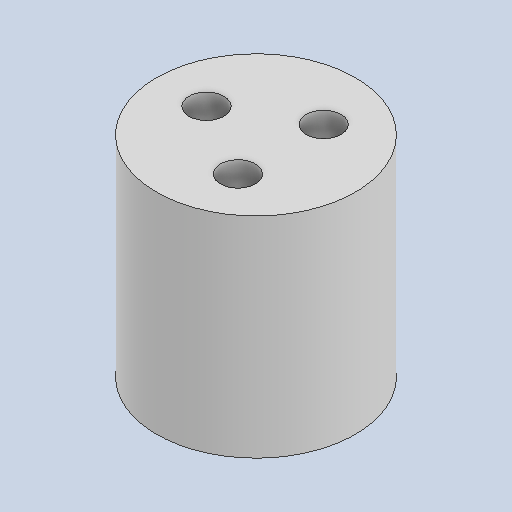
# Autodesk Inventor part: thigh_joint
Saved by Autodesk Inventor 2025.2 (Build 292293000, 293)
## iProperties
Created: 2025-04-10
Part Number: thigh_joint
Material: Generic
Document SubType Name: Modeling
Designer: Bruno
Density: 1 g/cm^3
Appearance: Default
Author: Bruno
Autodesk Inventor part; units mm, degrees
ref_plane "YZ Plane" through (0, 0, 0) normal (1, 0, 0) x (0, 1, 0)
ref_plane "XZ Plane" through (0, 0, 0) normal (0, 1, 0) x (-1, 0, 0)
ref_plane "XY Plane" through (0, 0, 0) normal (0, 0, 1) x (1, 0, 0)
sketch "Sketch1" plane through (0, 0, 0) normal (0, 1, 0) x (-1, 0, 0)
  circle A0 centre (0, 0) radius 8.5213
  dimension "d0" = 17.0425
  constraints: 1 centre point, 1 coincident
  measures "d0" diameter of A0
extrude "Extrusion1" add sketch "Sketch1" along normal blind 18
sketch "Sketch2" plane through (0, 18, 0) normal (0, 1, 0) x (1, 0, 0)
  circle A0 centre (0, 0) radius 8.5213 projected
  circle A1 centre (0, 0) radius 4.25 construction
  circle A2 centre (-4.25, 0) radius 1.5
  circle A3 centre (2.125, -3.6806) radius 1.5
  circle A4 centre (2.125, 3.6806) radius 1.5
  dimension "d3" = 8.5
  dimension "d4" = 3
  dimension "d7" = 360
  constraints: 3 centre point, 2 horizontal alignment, 1 coincident, 9 other
  measures "d4" diameter of A2
extrude "Extrusion2" cut sketch "Sketch2" against normal through all contours A2 | A3 | A4
body "Solid1"
